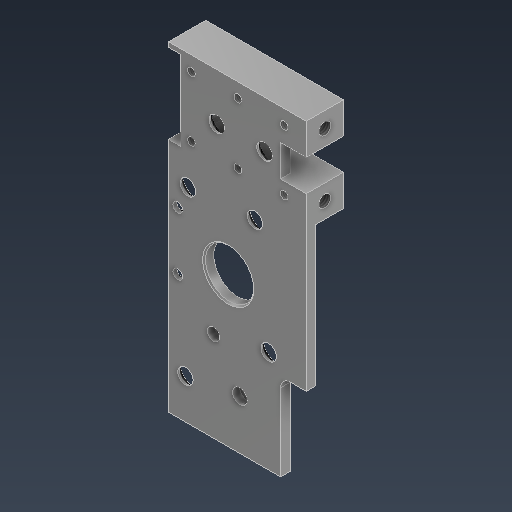
# Autodesk Inventor part: LeftGearboxCoverr
Saved by Autodesk Inventor 2027.1 (Build 311270010, 270A)
## iProperties
Created: 2026-04-13
Part Number: LeftGearboxCoverr
Material: Steel, Alloy
Document SubType Name: Modeling
Designer: szymo
Density: 7.73 g/cm^3
Appearance: Nylon 6(1)
Mass: 36.7541 g
Surface Area: 48.2465 cm^2
Volume: 4.75473 cm^3
Author: szymo
Autodesk Inventor part; units mm, degrees
ref_plane "YZ Plane" through (0, 0, 0) normal (1, 0, 0) x (0, 1, 0)
sketch "Sketch1" plane through (0, 0, 0) normal (0, 0, 1) x (1, 0, 0)
  circle A0 centre (14.75, -56.1789) radius 14.75 construction
  circle A1 centre (12.35, -35.5681) radius 5
  circle A2 centre (14.75, -14.75) radius 14.75 construction
  line L0 (23.2, -66.4289) -> (0, -66.4289)
  line L1 (0, -66.4289) -> (0, 0)
  line L2 (0, 0) -> (28.5, 0)
  line L3 (28.5, 0) -> (28.5, -19.5)
  line L4 (2.5, -1) -> (2.5, -9.4261)
  line L5 (2.5, -1) -> (1, -1)
  line L6 (1, -1) -> (1, -1)
  line L7 (1, -1) -> (0, -1)
  line L8 (2.5, -9.4261) -> (2.5, -17.5)
  line L9 (2.5, -17.5) -> (1, -17.5)
  line L10 (1, -17.5) -> (1, -17.5)
  line L11 (1, -17.5) -> (0, -17.5)
  line L12 (7.8575, -6.5) -> (28.5, -6.5)
  line L13 (7.8575, -6.5) -> (2.5, -6.5)
  line L14 (2.5, -13) -> (28.5, -13)
  line L15 (0, -19.5) -> (28.5, -19.5)
  circle A3 centre (14.75, -56.1789) radius 1.5
  circle A4 centre (9.3012, -47.7937) radius 1.25
  line L16 (23.2, -13) -> (23.2, -6.5)
  circle A5 centre (14.75, -56.1789) radius 14.75 projected
  circle A6 centre (14.75, -56.1789) radius 14.25 projected
  circle A7 centre (14.75, -14.75) radius 5.5 projected
  circle A8 centre (14.75, -14.75) radius 14.75 projected
  circle A9 centre (14.75, -14.75) radius 14.25 projected
  circle A10 centre (12.35, -35.5681) radius 5 projected
  circle A11 centre (12.35, -35.5681) radius 5.4 projected
  line L17 (1.5, -1) -> (1.5, -17) projected
  line L18 (2.5, -1) -> (1.5, -1) projected
  line L19 (2.5, -17) -> (2.5, -1) projected
  line L20 (2.5, -17) -> (1.5, -17) projected
  circle A12 centre (9.3012, -47.7937) radius 1.25 projected
  arc A13 (10.3711, -45.1522) -> (10.3563, -43.7284) centre (6.7284, -44.4781) ccw projected
  arc A14 (10.7068, -45.3144) -> (10.3711, -45.1522) centre (9.3012, -47.7937) ccw projected
  arc A15 (11.8317, -44.4416) -> (10.7068, -45.3144) centre (13.4977, -47.7504) ccw projected
  arc A16 (12.2476, -44.8006) -> (11.8317, -44.4416) centre (9.3012, -47.7937) ccw projected
  arc A17 (11.5486, -46.041) -> (12.2476, -44.8006) centre (8.7309, -43.6359) ccw projected
  arc A18 (11.7581, -46.3493) -> (11.5486, -46.041) centre (9.3012, -47.7937) ccw projected
  arc A19 (13.1688, -46.156) -> (11.7581, -46.3493) centre (12.9572, -49.8545) ccw projected
  arc A20 (13.3494, -46.6748) -> (13.1688, -46.156) centre (9.3012, -47.7937) ccw projected
  arc A21 (12.1238, -47.3995) -> (13.3494, -46.6748) centre (10.8863, -43.9078) ccw projected
  arc A22 (12.1511, -47.7713) -> (12.1238, -47.3995) centre (9.3012, -47.7937) ccw projected
  arc A23 (13.4695, -48.3092) -> (12.1511, -47.7713) centre (11.437, -51.4064) ccw projected
  arc A24 (13.3665, -48.8488) -> (13.4695, -48.3092) centre (9.3012, -47.7937) ccw projected
  arc A25 (11.9428, -48.8636) -> (13.3665, -48.8488) centre (12.6169, -45.2209) ccw projected
  arc A26 (11.7805, -49.1993) -> (11.9428, -48.8636) centre (9.3012, -47.7937) ccw projected
  arc A27 (12.6533, -50.3242) -> (11.7805, -49.1993) centre (9.3445, -51.9902) ccw projected
  arc A28 (12.2943, -50.7401) -> (12.6533, -50.3242) centre (9.3012, -47.7937) ccw projected
  arc A29 (11.0539, -50.041) -> (12.2943, -50.7401) centre (13.459, -47.2234) ccw projected
  arc A30 (10.7456, -50.2506) -> (11.0539, -50.041) centre (9.3012, -47.7937) ccw projected
  arc A31 (10.9389, -51.6612) -> (10.7456, -50.2506) centre (7.2404, -51.4496) ccw projected
  arc A32 (10.4201, -51.8419) -> (10.9389, -51.6612) centre (9.3012, -47.7937) ccw projected
  arc A33 (9.6954, -50.6163) -> (10.4201, -51.8419) centre (13.1871, -49.3787) ccw projected
  arc A34 (9.3236, -50.6436) -> (9.6954, -50.6163) centre (9.3012, -47.7937) ccw projected
  arc A35 (8.7858, -51.9619) -> (9.3236, -50.6436) centre (5.6886, -49.9294) ccw projected
  arc A36 (8.2461, -51.859) -> (8.7858, -51.9619) centre (9.3012, -47.7937) ccw projected
  arc A37 (8.2313, -50.4352) -> (8.2461, -51.859) centre (11.874, -51.1093) ccw projected
  arc A38 (7.8957, -50.273) -> (8.2313, -50.4352) centre (9.3012, -47.7937) ccw projected
  arc A39 (6.7707, -51.1458) -> (7.8957, -50.273) centre (5.1047, -47.837) ccw projected
  arc A40 (6.3548, -50.7868) -> (6.7707, -51.1458) centre (9.3012, -47.7937) ccw projected
  arc A41 (7.0539, -49.5464) -> (6.3548, -50.7868) centre (9.8715, -51.9515) ccw projected
  arc A42 (6.8443, -49.2381) -> (7.0539, -49.5464) centre (9.3012, -47.7937) ccw projected
  arc A43 (5.4337, -49.4314) -> (6.8443, -49.2381) centre (5.6453, -45.7329) ccw projected
  arc A44 (5.253, -48.9126) -> (5.4337, -49.4314) centre (9.3012, -47.7937) ccw projected
  arc A45 (6.4786, -48.1879) -> (5.253, -48.9126) centre (7.7162, -51.6796) ccw projected
  arc A46 (6.4513, -47.8161) -> (6.4786, -48.1879) centre (9.3012, -47.7937) ccw projected
  arc A47 (5.133, -47.2782) -> (6.4513, -47.8161) centre (7.1655, -44.181) ccw projected
  arc A48 (5.2359, -46.7386) -> (5.133, -47.2782) centre (9.3012, -47.7937) ccw projected
  arc A49 (6.6597, -46.7238) -> (5.2359, -46.7386) centre (5.9856, -50.3665) ccw projected
  arc A50 (6.8219, -46.3881) -> (6.6597, -46.7238) centre (9.3012, -47.7937) ccw projected
  arc A51 (5.9491, -45.2632) -> (6.8219, -46.3881) centre (9.2579, -43.5972) ccw projected
  arc A52 (6.3081, -44.8473) -> (5.9491, -45.2632) centre (9.3012, -47.7937) ccw projected
  arc A53 (7.5485, -45.5464) -> (6.3081, -44.8473) centre (5.1434, -48.364) ccw projected
  arc A54 (7.8569, -45.3368) -> (7.5485, -45.5464) centre (9.3012, -47.7937) ccw projected
  arc A55 (7.6635, -43.9262) -> (7.8569, -45.3368) centre (11.362, -44.1378) ccw projected
  arc A56 (8.1823, -43.7455) -> (7.6635, -43.9262) centre (9.3012, -47.7937) ccw projected
  arc A57 (8.907, -44.9711) -> (8.1823, -43.7455) centre (5.4153, -46.2087) ccw projected
  arc A58 (9.2788, -44.9438) -> (8.907, -44.9711) centre (9.3012, -47.7937) ccw projected
  arc A59 (9.8167, -43.6255) -> (9.2788, -44.9438) centre (12.9139, -45.658) ccw projected
  arc A60 (10.3563, -43.7284) -> (9.8167, -43.6255) centre (9.3012, -47.7937) ccw projected
  circle A61 centre (23.925, -15.5491) radius 0.75
  circle A62 centre (4.725, -15.5491) radius 0.75
  circle A63 centre (14.325, -3) radius 0.75
  line L21 (23.2, -19.55) -> (23.2, -66.4289)
  circle A64 centre (12.35, -35.5681) radius 15
  line L22 (23.2, -48.4289) -> (28.5, -48.4289)
  line L23 (28.5, -48.4289) -> (28.5, -19.5)
  line L24 (23.2, -9.3) -> (2.5, -9.3)
  circle A65 centre (23.925, -3.0509) radius 0.75
  circle A66 centre (4.725, -3.0509) radius 0.75
  circle A67 centre (14.325, -15.6) radius 0.75
  line L25 (26.7043, -21.0474) -> (25.0617, -19.4049) projected
  arc A68 (25.0617, -19.4049) -> (23.4815, -19.6245) centre (24.3546, -20.112) ccw projected
  arc A69 (19.6245, -23.4815) -> (23.4815, -19.6245) centre (14.75, -14.75) ccw projected
  arc A70 (19.6245, -23.4815) -> (19.4049, -25.0617) centre (20.112, -24.3546) ccw projected
  line L26 (19.4049, -25.0617) -> (21.0474, -26.7043) projected
  arc A71 (21.0474, -26.7043) -> (22.2832, -26.846) centre (21.7545, -25.9972) ccw projected
  arc A72 (2.654, -7.2168) -> (22.2832, -26.846) centre (14.75, -14.75) ccw projected
  arc A73 (2.654, -7.2168) -> (2.7957, -8.4526) centre (3.5028, -7.7455) ccw projected
  line L27 (2.7957, -8.4526) -> (4.4383, -10.0951) projected
  arc A74 (4.4383, -10.0951) -> (6.0185, -9.8755) centre (5.1454, -9.388) ccw projected
  arc A75 (9.8755, -6.0185) -> (6.0185, -9.8755) centre (14.75, -14.75) ccw projected
  arc A76 (9.8755, -6.0185) -> (10.0951, -4.4383) centre (9.388, -5.1454) ccw projected
  line L28 (10.0951, -4.4383) -> (8.4526, -2.7957) projected
  arc A77 (8.4526, -2.7957) -> (7.2168, -2.654) centre (7.7455, -3.5028) ccw projected
  arc A78 (26.846, -22.2832) -> (7.2168, -2.654) centre (14.75, -14.75) ccw projected
  arc A79 (26.846, -22.2832) -> (26.7043, -21.0474) centre (25.9972, -21.7545) ccw projected
  point P0 (6.8877, -8.4575)
  point P1 (5.3877, -11.0556)
  point P2 (24.0123, -18.3444)
  point P3 (22.5123, -20.9425)
  point P4 (2.5, -13)
  point P5 (5.7809, -45.1056)
  point P6 (6.4132, -44.6221)
  point P7 (7.3754, -43.9855)
  point P8 (8.0758, -43.5885)
  point P9 (23.1, -19.5)
  point P10 (0.2586, -17.5)
  point P11 (0, -14.75)
  dimension "d23" = 3
  dimension "d26" = 2.5
  dimension "d32" = 19.5
  dimension "d33" = 6.5
  dimension "d34" = 0.5
  dimension "d35" = 0.5
  dimension "d36" = 0
  dimension "d37" = 0
  dimension "d42" = 4.5
  dimension "d43" = 6.5
  dimension "d58" = 1
  dimension "d59" = 6.3
  dimension "d79" = 30
  dimension "d80" = 18
  dimension "d81" = 3.15
  constraints: 42 end point, 13 point on line, 12 centre point, 12 coincident, 12 perpendicular, 6 symmetric about line, 5 horizontal, 5 tangent, 3 parallel, 2 collinear, 1 vertical, 16 other
  measures "d23" diameter of A3
  measures "d26" diameter of A4
  measures "d32" distance between parallel lines of L15 L2
  measures "d33" distance between parallel lines of L15 L14
  measures "d34" distance between parallel lines of L9 L20
  measures "d35" distance between parallel lines of L10 L17
  measures "d36" distance between parallel lines of L11 L9
  measures "d37" distance between parallel lines of L7 L5
  measures "d42" distance edge to line of A0 L0
  measures "d43" distance between parallel lines of L12 L2
  measures "d58" distance edge to line of A2 L3
  measures "d59" distance edge to line of A2 L21
  measures "d79" diameter of A64
  measures "d80" distance between parallel lines of L0 L22
  measures "d81" distance edge to line of A67 L15
extrude "Extrusion3" add sketch "Sketch1" against normal blind 2 contours L0 A6 A64 A45 A44 A43 A41 A40 A39 A38 A37 A36 A35 A34 A33 A32 A31 A29 A28 L21 | L0 A5 A64 A6 | L21 A64 A6 L22 | L0 L1 A5 | A64 A5 L21 A6 | A6 L21 A64 A28 A27 A26 A25 A24 A23 A22 A21 A20 A19 A18 A17 A16 A15 A14 A13 A60 A59 A58 A57 A56 A55 A54 A53 A52 A51 A50 A49 A48 A47 A46 A45 | L21 A6 A64 | A6 A64 A5 L22 | L1 A64 A5 | L21 A5 A64 A6 | A64 L1 A8 L21 A5 | A64 A43 A44 A45 | A45 A46 A47 A48 A49 A50 A51 A52 A53 A54 A55 A56 A57 A58 A59 A60 A13 A14 A15 A16 A17 A18 A19 A20 A21 A22 A23 A24 A25 A26 A27 A28 A64 A29 A30 A31 A41 A42 A43 | A28 A29 A64 | A5 A64 A8 L23 L22 | L21 A8 A64 A5 | A43 A42 A41 A64 | A64 A31 A30 A29 | L1 L15 A8 A64 | L21 A9 A64 A8 | A8 A64 A9 L21 | A64 A31 A32 A33 A34 A35 A36 A37 A38 A39 A40 A41 | A8 A64 A9 L15 L23 | L1 L11 A8 L15 | A8 L15 A9 A64 | L21 A64 A9 | A9 A71 L26 A70 A69 A64 L21 | L15 A9 L3 | A8 L11 A9 L15 | A64 A69 A70 L26 A71 A9 | A9 L15 A7 A68 A69 A64 | A64 L21 A69 A68 L15 L25 A79 A9 | A64 A69 L21 | A9 L15 L25 A68 A7 L14 L3 | A9 A79 L25 L15 | A9 L11 L9 L8 L14 A7 L15 | L12 A8 A65 L2 L3 | L12 A9 A65 A8 | L15 A68 L25 | L1 L2 A8 A66 L13 L4 L5 L7 | A7 L14 L15 | L15 A7 | L12 A75 A76 L28 A77 A9 A65 | A65 A9 A8 | A8 A65 | L14 A7 L24 L16 | A8 L13 A9 L4 | L4 L13 A8 | A7 L24 L14 | L14 L8 L4 L24 L27 A74 A75 A7 | A8 A65 A9 L13 A66 | L16 L24 A7 A75 L12 | A65 A9 | A9 A73 L27 L24 L4 | A7 L24 | A66 A8 | A8 A66 | A75 L24 L27 A73 A9 L13 L12 | L12 L13 A9 A77 L28 A76 A75 | A75 A74 L27 L24 | A3 | A4 | A11 | A61 | A62 | A63 | A67
ref_plane "Work Plane1" through (1, -19, -6.7) normal (0, 0, 1) x (1, 0, 0)
ref_plane "Work Plane2" through (1, -19, -7.7) normal (0, 0, 1) x (1, 0, 0)
extrude "Extrusion4" add sketch "Sketch1" against normal up to surface (7.7 mm away) contours L1 L11 A8 L15 | L15 A9 L3 | A8 L11 A9 L15 | A9 L15 L25 A68 A7 L14 L3 | A9 L11 L9 L8 L14 A7 L15 | L12 A8 A65 L2 L3 | L12 A9 A65 A8 | L15 A68 L25 | L1 L2 A8 A66 L13 L4 L5 L7 | A7 L14 L15 | L12 A75 A76 L28 A77 A9 A65 | A65 A9 A8 | A8 A65 | A8 A65 A9 L13 A66 | A65 A9 | A66 A8 | A8 A66 | L12 L13 A9 A77 L28 A76 A75 | A61 | A62 | A63 | A67
hole "Hole1" at (23.925, -15.5491, 0) at (4.725, -15.5491, 0) at (14.325, -3, 0) at (14.325, -15.6, 0) at (4.725, -3.0509, 0) at (23.925, -3.0509, 0) direction (0, 0, -1) diameter 1.567 end through all thread size "M2x0.4" class "6H" standard "ISO Metric profile"
extrude "Extrusion5" cut sketch "Sketch1" against normal blind 1.5 contours A3 | A4
sketch "Sketch2" plane through (0, 0, -2) normal (0, 0, -1) x (-1, 0, 0)
  line L0 (-2.5, -17.5) -> (0, -17.5) projected
  line L1 (-2.5, -1) -> (-2.5, -17.5) projected
  line L2 (0, -1) -> (-2.5, -1) projected
  line L3 (0, -17.5) -> (0, -66.4289) projected
  line L4 (-28.4, 0) -> (0, 0) projected
  line L5 (-28.4, -6.5) -> (-28.4, 0) projected
  line L6 (-23.2, -6.5) -> (-28.4, -6.5) projected
  line L7 (-23.2, -66.4289) -> (-23.2, -6.5) projected
  line L8 (0, -66.4289) -> (-23.2, -66.4289) projected
  line L9 (0, 0) -> (0, -1) projected
  arc A0 (-16.8677, -44.1456) -> (-16.9976, -51.1591) centre (-9.3012, -47.7937) ccw projected
  arc A1 (-4.2588, -41.0755) -> (-16.8677, -44.1456) centre (-12.35, -35.2722) ccw projected
  circle A2 centre (-9.0931, -61.8357) radius 2.25 projected
  circle A3 centre (-1.9, -28.7694) radius 0.7 projected
  circle A4 centre (-1.9, -40.729) radius 0.7 projected
  arc A5 (-9.25, -56.1935) -> (-4.2588, -41.0755) centre (-9.3012, -47.7937) ccw projected
  circle A6 centre (-17.8716, -23) radius 1.2295 projected
  circle A7 centre (-9.95, -9.75) radius 1.2295 projected
  circle A8 centre (-19.95, -9.75) radius 1.2295 projected
  circle A9 centre (-20.7179, -45.3169) radius 1.2295 projected
  circle A10 centre (-4, -24.0883) radius 1.2295 projected
  circle A11 centre (-3.5, -58.1839) radius 1.2295 projected
  circle A12 centre (-20.3569, -49.9802) radius 2.25 projected
  circle A13 centre (-20.4069, -50.522) radius 2.25 projected
  arc A14 (-16.9976, -51.1591) -> (-9.25, -56.1935) centre (-14.75, -56.1789) ccw projected
  point P0 (-19.873, -45.2549)
  point P1 (-3.5, -57.971)
  point P2 (-4, -24.0349)
  point P3 (-17.9752, -23)
  point P4 (-19.85, -9.75)
  point P5 (-9.85, -9.75)
  point P6 (-19.873, -45.2549)
  point P7 (-20.3569, -49.9802)
  point P8 (-19.873, -45.2549)
  point P9 (-19.873, -45.2549)
  point P10 (-9.002, -47.4193)
  point P11 (-12.35, -35.2722)
  point P12 (-14.7, -55.6371)
  point P13 (-12.35, -35.2722)
  point P14 (-14.7, -55.6371)
  point P15 (-12.35, -35.2722)
  point P16 (-14.7, -55.6371)
  point P17 (-19.873, -45.2549)
  point P18 (-9.002, -47.4193)
  point P19 (-14.7, -55.6371)
  point P20 (-19.873, -45.2549)
  point P21 (-21.2554, -47.9174)
  point P22 (-12.35, -35.2722)
  point P23 (-14.7, -55.6371)
  point P24 (-19.0589, -48.1424)
  point P25 (-19.873, -45.2549)
  point P26 (-14.7, -55.6371)
  point P27 (-20.3569, -49.9802)
  point P28 (-19.873, -45.2549)
  point P29 (-12.35, -35.2722)
  point P30 (-19.873, -45.2549)
  point P31 (-14.7, -55.6371)
  point P32 (-20.3569, -49.9802)
  point P33 (-19.873, -45.2549)
  point P34 (-12.35, -35.2722)
  point P35 (-19.873, -45.2549)
  point P36 (-14.7, -55.6371)
  point P37 (-20.3569, -49.9802)
  point P38 (-19.873, -45.2549)
  point P39 (-12.35, -35.2722)
  point P40 (-19.873, -45.2549)
  point P41 (-14.7, -55.6371)
  point P42 (-20.3569, -49.9802)
  point P43 (-19.873, -45.2549)
  point P44 (-12.35, -35.2722)
  point P45 (-19.873, -45.2549)
  point P46 (-14.7, -55.6371)
  point P47 (-20.3569, -49.9802)
  point P48 (-19.873, -45.2549)
  point P49 (-12.35, -35.2722)
  point P50 (-19.873, -45.2549)
  point P51 (-20.3569, -49.9802)
  point P52 (-9.002, -47.4193)
  point P53 (-12.35, -35.2722)
  point P54 (-9.002, -47.4193)
  point P55 (-9.002, -47.4193)
  point P56 (-9.002, -47.4193)
  point P57 (-9.002, -47.4193)
  point P58 (-9.002, -47.4193)
  point P59 (-9.002, -47.4193)
  point P60 (-9.002, -47.4193)
  point P61 (-9.002, -47.4193)
  point P62 (-9.002, -47.4193)
  point P63 (-9.002, -47.4193)
  point P64 (-9.002, -47.4193)
  point P65 (-9.002, -47.4193)
  point P66 (-9.002, -47.4193)
  point P67 (-9.002, -47.4193)
  point P68 (-9.002, -47.4193)
  point P69 (-9.002, -47.4193)
  point P70 (-9.002, -47.4193)
  point P71 (-9.002, -47.4193)
  point P72 (-9.002, -47.4193)
  point P73 (-9.002, -47.4193)
  point P74 (-9.002, -47.4193)
  point P75 (-9.002, -47.4193)
  point P76 (-9.002, -47.4193)
  point P77 (-9.002, -47.4193)
  point P78 (-9.002, -47.4193)
  point P79 (-9.002, -47.4193)
  point P80 (-9.002, -47.4193)
  point P81 (-9.002, -47.4193)
  point P82 (-9.002, -47.4193)
  point P83 (-9.002, -47.4193)
  constraints: 1 other
hole "Hole2" at (20.7179, -45.3169, -2) at (3.5, -58.1839, -2) at (4, -24.0883, -2) at (17.8716, -23, -2) at (19.85, -9.75, -2) at (9.95, -9.75, -2) direction (0, 0, 1) diameter 3.2 depth 5 countersink diameter 6.5 countersink angle 90 clearance for "Countersunk Flat Head Screw ISO 2009/7046" size "M3" standard "ISO"
sketch "Sketch3" plane through (28.5, -6.5, 0) normal (1, 0, 0) x (0, 0, -1)
  line L0 (0, 0) -> (0, 6.5) projected
  line L1 (7.7, 6.5) -> (7.7, 0) projected
  line L2 (0, 6.5) -> (7.7, 6.5) projected
  line L3 (0, -6.5) -> (0, 0) projected
  line L4 (0, 0) -> (7.7, 6.5)
  line L5 (0, 6.5) -> (7.7, 0)
  line L6 (0, 0) -> (7.7, 0) projected
  line L7 (0, -13) -> (7.7, -6.5)
  line L8 (7.7, -13) -> (0, -6.5)
  point P0 (0, 6.5)
  point P1 (3.85, 3.25)
  point P2 (3.85, -9.75)
  constraints: 8 end point, 2 midpoint
hole "Hole3" at (28.5, -3.25, -3.85) at (28.5, -16.25, -3.85) direction (-1, 0, 0) diameter 2.459 depth 10 thread size "M3x0.5" class "6H" standard "ISO Metric profile"
sketch "Sketch4" plane through (0, 0, -2) normal (0, 0, -1) x (-1, 0, 0)
  circle A0 centre (-1.9, -40.729) radius 0.7 projected
  circle A1 centre (-1.9, -28.7694) radius 0.7 projected
  circle A2 centre (-1.9, -40.729) radius 2
  circle A3 centre (-1.9, -28.7694) radius 2
  line L0 (-1.9, -42.729) -> (0.1, -42.729)
  line L1 (0.1, -42.729) -> (0.1, -38.729)
  line L2 (0.1, -38.729) -> (-1.9, -38.729)
  line L3 (-1.9, -38.729) -> (-1.9, -42.729)
  line L4 (-1.9, -26.7694) -> (0.1, -26.7694)
  line L5 (0.1, -26.7694) -> (0.1, -30.7694)
  line L6 (0.1, -30.7694) -> (-1.9, -30.7694)
  line L7 (-1.9, -30.7694) -> (-1.9, -26.7694)
  point P0 (0, 0)
  point P1 (-1.9, -38.729)
  dimension "d60" = 4
  dimension "d61" = 4
  constraints: 16 end point, 5 horizontal, 4 parallel, 2 coincident, 2 perpendicular, 2 vertical, 1 point on line, 6 other
extrude "Extrusion7" cut sketch "Sketch4" against normal blind 1.2
sketch "Sketch5" plane through (0, 0, -2) normal (0, 0, -1) x (-1, 0, 0)
  arc A0 (-1.9, -38.729) -> (-1.9, -42.729) centre (-1.9, -40.729) ccw projected
  arc A1 (-1.9, -26.7694) -> (-1.9, -30.7694) centre (-1.9, -28.7694) ccw projected
  point P0 (0, 0)
hole "Hole4" at (1.9, -40.729, -2) at (1.9, -28.7694, -2) direction (0, 0, 1) diameter 2 end through all clearance for "Countersunk Flat Head Screw ISO 2009/7046" size "M2" standard "ISO"
chamfer "Chamfer2" distance 2 angle 25 2 edges at (2.5, -6.5, -4.85) (2.5, -13, -4.85) measured on face at (2.5, -13.5, -4.85) measured on face at (2.5, -6, -4.85)
fillet "Fillet1" radius 4 4 edges at (2.5, -15, -4.85) (3.4326, -13, -4.85) (3.4326, -6.5, -4.85) (2.5, -4.5, -4.85)
fillet "Fillet3" radius 2 1 edges at (23.2, -48.4289, -1)
chamfer "Chamfer3" distance 0.3 angle 45 1 edges at (7.35, -35.5681, 0)
body "Solid3"
